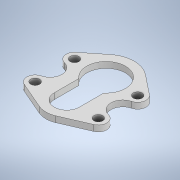
# Autodesk Inventor part: Part9
Saved by Autodesk Inventor 2021 (Build 250183000, 183)
## iProperties
Created: 2022-04-24
Part Number: Part9
Material: Generic
Document SubType Name: Modeling
Designer: hp
Density: 1 g/cm^3
Appearance: Default
Author: hp
Autodesk Inventor part; units mm, degrees
ref_plane "YZ Plane" through (0, 0, 0) normal (1, 0, 0) x (0, 1, 0)
ref_plane "XZ Plane" through (0, 0, 0) normal (0, 1, 0) x (-1, 0, 0)
ref_plane "XY Plane" through (0, 0, 0) normal (0, 0, 1) x (1, 0, 0)
sketch "Sketch1" plane through (0, 0, 0) normal (0, 1, 0) x (-1, 0, 0)
  arc A0 (13.8679, 98.1353) -> (0, 101) centre (0, 66) ccw
  arc A1 (0, -47) -> (29.2642, -36.7778) centre (0, 0) ccw
  arc A2 (56.3704, 52.4118) -> (58.5472, 78.8541) centre (53, 66) ccw
  arc A3 (61.717, -10.9551) -> (56.3704, 13.5882) centre (53, 0) ccw
  line L0 (13.8679, 98.1353) -> (58.5472, 78.8541)
  line L1 (61.717, -10.9551) -> (29.2642, -36.7778)
  arc A4 (56.3704, 52.4118) -> (56.3704, 13.5882) centre (61.1854, 33) ccw
  line L2 (0, 101) -> (0, -47)
  arc A5 (21, 66) -> (0, 87) centre (0, 66) ccw
  arc A6 (0, -32.5) -> (21, 24.8042) centre (0, 0) ccw
  line L3 (21, 66) -> (21, 24.8042)
  circle A7 centre (53, 66) radius 7.5
  circle A8 centre (53, 0) radius 7.5
  arc A9 (0, 101) -> (-13.8679, 98.1353) centre (0, 66) ccw
  arc A10 (-29.2642, -36.7778) -> (0, -47) centre (0, 0) ccw
  arc A11 (-58.5472, 78.8541) -> (-56.3704, 52.4118) centre (-53, 66) ccw
  arc A12 (-56.3704, 13.5882) -> (-61.717, -10.9551) centre (-53, 0) ccw
  line L4 (-13.8679, 98.1353) -> (-58.5472, 78.8541)
  line L5 (-61.717, -10.9551) -> (-29.2642, -36.7778)
  arc A13 (-56.3704, 13.5882) -> (-56.3704, 52.4118) centre (-61.1854, 33) ccw
  arc A14 (0, 87) -> (-21, 66) centre (0, 66) ccw
  arc A15 (-21, 24.8042) -> (0, -32.5) centre (0, 0) ccw
  line L6 (-21, 66) -> (-21, 24.8042)
  circle A16 centre (-53, 66) radius 7.5
  circle A17 centre (-53, 0) radius 7.5
  dimension "d0" = 94
  dimension "d1" = 70
  dimension "d2" = 66
  dimension "d3" = 0
  dimension "d4" = 28
  dimension "d5" = 28
  dimension "d6" = 53
  dimension "d7" = 0
  dimension "d8" = 0
  dimension "d9" = 66
  dimension "d10" = 40
  dimension "d11" = 42
  dimension "d12" = 65
  dimension "d13" = 15
  dimension "d14" = 15
  constraints: 28 point on circle, 18 centre point, 14 end point, 13 symmetric about line, 8 coincident, 7 tangent, 2 point on line, 2 vertical, 9 other
  measures "d0" diameter of A1
  measures "d1" diameter of A0
  measures "d2" distance of A0.centre A1.centre
  measures "d3" distance of A1.centre point (0, 0)
  measures "d4" diameter of A2
  measures "d5" diameter of A3
  measures "d6" distance of A0.centre A2.centre
  measures "d7" horizontal distance of A3.centre A2.centre
  measures "d8" vertical distance of point (0, 0) A3.centre
  measures "d9" distance of A3.centre A2.centre
  measures "d10" diameter of A4
  measures "d11" diameter of A5
  measures "d12" diameter of A6
  measures "d13" diameter of A7
  measures "d14" diameter of A8
extrude "Extrusion1" add sketch "Sketch1" along normal blind 10 contours L0 A2 A4 A3 L1 A1 L2 A6 L3 A5 A0 | L2 A14 L6 A15 A10 L5 A12 A13 A11 L4 A9
equation "\"d5\" = d4"
body "Solid1"
